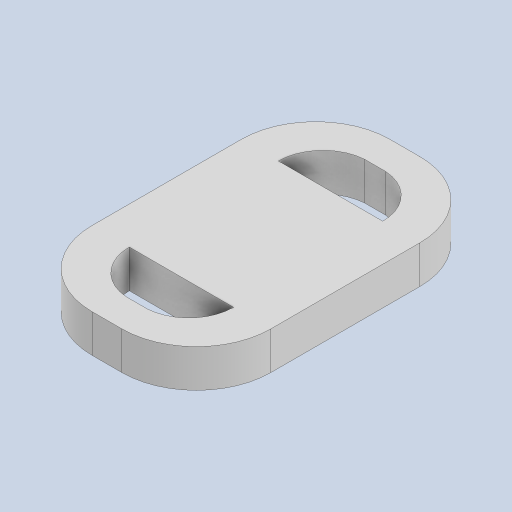
# Autodesk Inventor part: cuerpo
Saved by Autodesk Inventor 2024 (Build 280153000, 153)
## iProperties
Created: 2025-09-21
Part Number: cuerpo
Material: Genérico
Document SubType Name: Modeling
Designer: ANDRES
Density: 1 g/cm^3
Appearance: Valor por defecto
Author: ANDRES
Autodesk Inventor part; units mm, degrees
ref_plane "YZ Plane" through (0, 0, 0) normal (1, 0, 0) x (0, 1, 0)
ref_plane "XZ Plane" through (0, 0, 0) normal (0, 1, 0) x (-1, 0, 0)
ref_plane "XY Plane" through (0, 0, 0) normal (0, 0, 1) x (1, 0, 0)
sketch "Boceto1" plane through (0, 0, 0) normal (0, 1, 0) x (-1, 0, 0)
  line L0 (60, 50) -> (-60, 50)
  line L1 (-60, 50) -> (-60, -50)
  line L2 (-60, -50) -> (60, -50)
  line L3 (60, -50) -> (60, 50)
  line L4 (10, -100) -> (-10, -100)
  arc A0 (10, -100) -> (60, -50) centre (10, -50) ccw
  arc A1 (-60, -50) -> (-10, -100) centre (-10, -50) ccw
  line L5 (214.8695, 0) -> (-214.8695, 0) construction
  line L6 (-60, -50) -> (-60, 50)
  line L7 (60, 50) -> (60, -50)
  line L8 (10, 100) -> (-10, 100)
  arc A2 (60, 50) -> (10, 100) centre (10, 50) ccw
  arc A3 (-10, 100) -> (-60, 50) centre (-10, 50) ccw
  line L9 (35, -50) -> (-6.7192, -50)
  line L10 (35, -50) -> (35, -35.1557)
  arc A4 (7.1629, -79.9219) -> (35, -50) centre (5, -50) ccw
  line L11 (7.1629, -79.9219) -> (-7.1629, -79.9219)
  line L12 (0, -17.6821) -> (0, -145.6354) construction
  line L13 (-35, -50) -> (-35, -35.1557)
  arc A5 (-35, -50) -> (-7.1629, -79.9219) centre (-5, -50) ccw
  line L14 (-7.1629, -79.9219) -> (7.1629, -79.9219)
  line L15 (35, 50) -> (35, 35.1557)
  arc A6 (35, 50) -> (7.1629, 79.9219) centre (5, 50) ccw
  line L16 (7.1629, 79.9219) -> (-7.1629, 79.9219)
  line L17 (-35, 50) -> (-35, 35.1557)
  arc A7 (-7.1629, 79.9219) -> (-35, 50) centre (-5, 50) ccw
  point P0 (0, 0)
  point P1 (0, -100)
  point P2 (0, -50)
  point P3 (-60, 0)
  point P4 (0, 0)
  point P5 (-60, 0)
  point P6 (0, 50)
  point P7 (14.1404, -50)
  point P8 (0, -79.9219)
  point P9 (0, -81.6587)
  point P10 (35, 50)
  point P11 (-35, 50)
  point P12 (-7.1629, 79.9219)
  dimension "d0" = 120
  dimension "arco" = 50
  dimension "d2" = 50
  dimension "d3" = 200
  dimension "d5" = 70
  dimension "d6" = 30
  constraints: 36 end point, 22 symmetric about line, 16 point on circle, 9 midpoint, 8 centre point, 5 horizontal, 4 vertical alignment, 3 tangent, 2 horizontal alignment, 2 parallel, 2 vertical, 1 coincident, 1 perpendicular, 5 other
  measures "d0" distance from line of point (-60, 0) L3
  measures "arco" radius of A0
  measures "d2" radius of A1
  measures "d3" distance between parallel lines of L4 L8
  measures "d5" distance between parallel lines of L13 L10
  measures "d6" radius of A4
extrude "Extrusión1" add sketch "Boceto1" along normal blind 25.4 contours L3 L2 L1 L0 | L0 A6 L16 A7 A3 L8 A2 | A0 L4 A1 L2 A5 L11 A4
equation "\"d2\" = arco"
